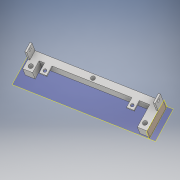
# Autodesk Inventor part: PC_top_piece
Saved by Autodesk Inventor 2017 (Build 210142000, 142)
## iProperties
Created: 2021-05-17
Part Number: PC_top_piece
Material: Generic
Document SubType Name: Modeling
Designer: Del
Density: 1 g/cm^3
Appearance: Default
Author: Del
Autodesk Inventor part; units mm, degrees
ref_plane "YZ Plane" through (0, 0, 0) normal (1, 0, 0) x (0, 1, 0)
ref_plane "XZ Plane" through (0, 0, 0) normal (0, 1, 0) x (-1, 0, 0)
ref_plane "XY Plane" through (0, 0, 0) normal (0, 0, 1) x (1, 0, 0)
sketch "Sketch1" plane through (0, 0, 0) normal (0, 0, 1) x (1, 0, 0)
  line L0 (-10.16, 7.62) -> (-15.748, 7.62)
  line L1 (-15.748, 7.62) -> (-15.748, 18.034)
  line L2 (-15.748, 18.034) -> (-23.368, 18.034)
  line L3 (-23.368, 18.034) -> (-23.368, 7.62)
  line L4 (-23.368, 7.62) -> (-105.283, 7.62)
  line L5 (-105.283, 7.62) -> (-105.283, 18.034)
  line L6 (-105.283, 18.034) -> (-112.903, 18.034)
  line L7 (-112.903, 18.034) -> (-112.903, 7.62)
  line L8 (-112.903, 7.62) -> (-123.571, 7.62)
  line L9 (-123.571, 7.62) -> (-123.571, 31.75)
  line L10 (-123.571, 31.75) -> (-133.731, 31.75)
  circle A0 centre (-109.093, 14.224) radius 1.778
  line L11 (-133.731, 31.75) -> (-133.731, 0)
  line L12 (-133.731, 0) -> (0, 0)
  circle A1 centre (-19.558, 14.224) radius 1.778
  line L13 (0, 0) -> (0, 20.32)
  line L14 (0, 20.32) -> (-10.16, 20.32)
  line L15 (-10.16, 20.32) -> (-10.16, 7.62)
  circle A2 centre (-128.143, 25.4) radius 2.413
  circle A3 centre (-63.5, 4.064) radius 2.413
  circle A4 centre (-5.6324, 15.2344) radius 2.413
  dimension "d22" = 20.32
  dimension "d39" = 4.826
  dimension "d40" = 4.826
  dimension "d41" = 4.826
  constraints: 32 end point, 5 centre point, 2 perpendicular, 1 vertical
  measures "d22" distance of L12.end L13.end
  measures "d39" diameter of A2
  measures "d40" diameter of A3
  measures "d41" diameter of A4
extrude "Extrusion2" add sketch "Sketch1" along normal blind 13.081 contours L15 L14 L13 L12 L11 L10 L9 L8 L7 L6 L5 L4 L3 L2 L1 L0 | A2 | A3 | A4
sketch "Sketch2" plane through (0, 0, 0) normal (0, 0, 1) x (1, 0, 0)
  line L0 (-10.16, 7.62) -> (-15.748, 7.62) projected
  line L1 (-12.954, 7.62) -> (-118.4109, 7.62)
  line L2 (-118.4109, 7.62) -> (-118.4109, 21.3127)
  line L3 (-118.4109, 21.3127) -> (-12.954, 21.3127)
  line L4 (-12.954, 21.3127) -> (-12.954, 7.62)
  point P0 (0, 0)
  constraints: 8 end point, 2 parallel, 1 horizontal, 1 midpoint, 1 perpendicular
extrude "Extrusion3" cut sketch "Sketch2" along normal blind 11.176
sketch "Sketch3" plane through (0, 0, 0) normal (1, 0, 0) x (0, 1, 0)
  line L0 (31.75, 13.081) -> (0, 13.081) projected
  line L1 (0.0413, 13.081) -> (0.0413, 28.575)
  line L2 (0.0413, 13.081) -> (15.5353, 13.081) construction
  line L3 (0.0413, 28.575) -> (10.2013, 28.575)
  line L4 (10.2013, 28.575) -> (10.2013, 13.081)
  circle A0 centre (5.1213, 24.8069) radius 1.778
  point P0 (0, 0)
  dimension "d28" = 15.494
  dimension "d29" = 90
  dimension "d30" = 10.16
  dimension "d31" = 3.556
  constraints: 8 end point, 4 perpendicular, 2 point on line, 1 centre point, 1 horizontal
  measures "d28" distance of L1.start L1.end
  measures "d29" angle of L2 L1
  measures "d30" distance of L1.end L3.end
  measures "d31" diameter of A0
extrude "Extrusion4" add sketch "Sketch3" against normal blind 2.032
ref_plane "Work Plane1" through (-133.731, 0, 0) normal (-1, 0, 0) x (0, 0, 1)
sketch "Sketch5" plane through (-133.731, 0, 0) normal (-1, 0, 0) x (0, 0, 1)
  line L0 (28.575, 10.2013) -> (13.081, 10.2013) projected
  line L1 (13.081, 0.0413) -> (28.575, 0.0413) projected
  line L2 (13.081, 10.2013) -> (28.575, 10.2013)
  line L3 (28.575, 10.2013) -> (28.575, 0.0413)
  line L4 (28.575, 0.0413) -> (13.081, 0.0413)
  line L5 (13.081, 0.0413) -> (13.081, 10.2013)
  circle A0 centre (24.7788, 5.1213) radius 1.778
  point P0 (0, 0)
  dimension "d36" = 3.556
  constraints: 8 end point, 2 parallel, 1 centre point, 1 horizontal, 1 perpendicular
  measures "d36" diameter of A0
extrude "Extrusion5" add sketch "Sketch5" against normal blind 2.032
ref_plane "Work Plane2" through (0, 0, 0) normal (0, 0, -1) x (-1, 0, 0)
sketch "Sketch6" plane through (0, 0, 0) normal (0, 0, -1) x (-1, 0, 0)
  circle A0 centre (5.588, 15.24) radius 2.413
  circle A1 centre (63.5, 4.0894) radius 2.286
  circle A2 centre (128.1176, 25.4) radius 2.413
  point P0 (0, 0)
  dimension "d43" = 4.826
  dimension "d44" = 4.572
  dimension "d45" = 4.826
  constraints: 3 centre point
  measures "d43" diameter of A0
  measures "d44" diameter of A1
  measures "d45" diameter of A2
extrude "Extrusion6" cut sketch "Sketch6" against normal blind 15.24
body "Solid2"
